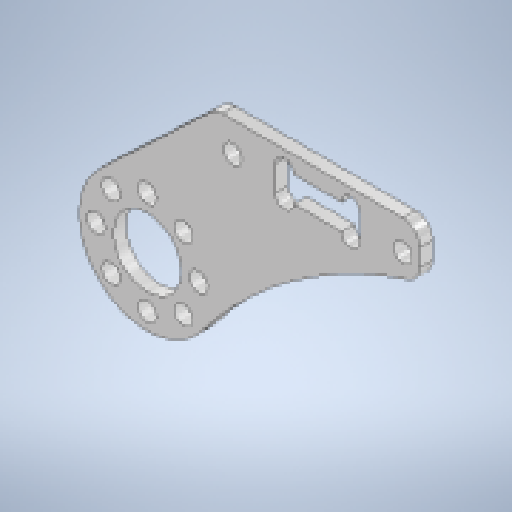
# Autodesk Inventor part: tesaki_new
Saved by Autodesk Inventor 2024 (Build 280153000, 153)
## iProperties
Created: 2023-12-16
Part Number: tesaki_new
Material: アルミニウム 2014-T4
Document SubType Name: Modeling
Designer: right
Density: 2.8 g/cm^3
Appearance: サテン
Mass: 2.30594 g
Surface Area: 15.3884 cm^2
Volume: 0.823551 cm^3
Author: right
Autodesk Inventor part; units mm, degrees
ref_plane "YZ Plane" through (0, 0, 0) normal (1, 0, 0) x (0, 1, 0)
ref_plane "XZ Plane" through (0, 0, 0) normal (0, 1, 0) x (-1, 0, 0)
ref_plane "XY Plane" through (0, 0, 0) normal (0, 0, 1) x (1, 0, 0)
sketch "スケッチ1" plane through (0, 0, 0) normal (0, 0, 1) x (1, 0, 0)
  circle A0 centre (8.8, 8.8) radius 8 projected
  circle A1 centre (2.8, 8.8) radius 0.825 projected
  circle A2 centre (4.5574, 4.5574) radius 0.825 projected
  circle A3 centre (8.8, 2.8) radius 0.825 projected
  circle A4 centre (13.0426, 4.5574) radius 0.825 projected
  circle A5 centre (14.8, 8.8) radius 0.825 projected
  circle A6 centre (13.0426, 13.0426) radius 0.825 projected
  circle A7 centre (8.8, 14.8) radius 0.825 projected
  circle A8 centre (4.5574, 13.0426) radius 0.825 projected
  circle A9 centre (8.8, 8.8) radius 4 projected
  circle A10 centre (8.8, 14.8) radius 1.1
  circle A11 centre (4.5574, 13.0426) radius 1.1
  circle A12 centre (2.8, 8.8) radius 1.1
  circle A13 centre (4.5574, 4.5574) radius 1.1
  circle A14 centre (8.8, 2.8) radius 1.1
  circle A15 centre (13.0426, 4.5574) radius 1.1
  circle A16 centre (14.8, 8.8) radius 1.1
  circle A17 centre (13.0426, 13.0426) radius 1.1
  line L0 (3.3206, 14.6289) -> (16.8, 27.3)
  line L1 (23.8, 25.3) -> (33.8, 25.3)
  line L2 (33.8, 25.3) -> (33.8, 22.3)
  line L3 (33.8, 22.3) -> (23.8, 22.3)
  line L4 (23.8, 22.3) -> (23.8, 25.3)
  circle A18 centre (24.9, 25.3) radius 1.1
  line L5 (28.8, 25.3) -> (28.8, 22.3) construction
  line L6 (28.8, 23.8) -> (23.8, 23.8) construction
  circle A19 centre (24.9, 22.3) radius 1.1
  circle A20 centre (32.7, 25.3) radius 1.1
  circle A21 centre (32.7, 22.3) radius 1.1
  circle A22 centre (38.8, 23.8) radius 1.1
  circle A23 centre (18.8, 23.8) radius 1.1
  line L7 (16.8, 27.3) -> (40.8, 27.3)
  line L8 (40.8, 27.3) -> (40.8, 21.8)
  arc A24 (40.8, 21.8) -> (15.1891, 3.9855) centre (55.1209, -26.1052) ccw
  point P0 (0, 0)
  point P1 (31.6, 22.3)
  point P2 (26, 22.3)
  point P3 (26, 25.3)
  point P4 (31.6, 25.3)
  dimension "d7" = 2.2
  dimension "d0" = 2.2
  dimension "d3" = 360
  dimension "d5" = 10
  dimension "d6" = 3
  dimension "d8" = 2.2
  dimension "d9" = 5
  dimension "d10" = 2
  dimension "d11" = 2
  dimension "d12" = 2
  dimension "d13" = 20
  dimension "d14" = 2
  dimension "d15" = 15
  dimension "d16" = 50
  constraints: 18 end point, 14 centre point, 4 midpoint, 4 point on circle, 4 symmetric about line, 2 horizontal, 2 parallel, 2 tangent, 1 coincident, 1 horizontal alignment, 1 perpendicular, 1 point on line, 1 vertical, 24 other
  measures "d0" diameter of A10
  measures "d5" distance of L2.end L3.end
  measures "d6" distance of L1.end L2.end
  measures "d8" diameter of A22
  measures "d9" distance from line of L4 A23.centre
  measures "d10" distance from line of L7 A20.centre
  measures "d11" distance from line of A22.centre L8
  measures "d12" horizontal distance of L0.end A23.centre
  measures "d13" horizontal distance of A9.centre L6.start
  measures "d14" horizontal distance of L8.end A22.centre
  measures "d15" vertical distance of A9.centre L6.start
  measures "d16" radius of A24
extrude "押し出し1" add sketch "スケッチ1" along normal blind 1.5 contours A0 | A0 L0 L7 L8 A24
fillet "フィレット1" radius 2 3 edges at (40.8, 27.3, 0.75) (40.8, 21.8, 0.75) (16.8, 27.3, 0.75)
sketch "スケッチ4" plane through (0, 0, 0) normal (0, 0, -1) x (-1, 0, 0)
  line L0 (-53.8, 25.3) -> (-43.8, 25.3)
  line L1 (-43.8, 25.3) -> (-43.8, 22.3)
  line L2 (-43.8, 22.3) -> (-53.8, 22.3)
  line L3 (-53.8, 22.3) -> (-53.8, 25.3)
  circle A0 centre (-38.8, 23.8) radius 1.1 projected
  circle A1 centre (-52.7, 25.3) radius 1.1
  line L4 (-48.8, 25.3) -> (-48.8, 23.8) construction
  line L5 (-48.8, 23.8) -> (-53.8, 23.8) construction
  circle A2 centre (-44.9, 25.3) radius 1.1
  circle A3 centre (-52.7, 22.3) radius 1.1
  circle A4 centre (-44.9, 22.3) radius 1.1
  arc A5 (-15.1891, 3.9855) -> (-39.4277, 21.3682) centre (-55.1209, -26.1052) ccw projected
  line L6 (-31.9466, 18.2) -> (-56.8, 18.2)
  line L7 (-56.8, 18.2) -> (-56.8, 27.3)
  line L8 (-38.8, 27.3) -> (-17.5925, 27.3) construction
  line L9 (-56.8, 27.3) -> (-38.8, 27.3)
  arc A6 (-16.2226, 26.7572) -> (-17.5925, 27.3) centre (-17.5925, 25.3) ccw projected
  line L10 (-38.8, 27.3) -> (-17.5925, 27.3) projected
  arc A7 (-38.8, 27.3) -> (-40.8, 25.3) centre (-38.8, 25.3) ccw projected
  line L11 (-40.8, 23.2671) -> (-40.8, 25.3) projected
  arc A8 (-40.8, 23.2671) -> (-39.4277, 21.3682) centre (-38.8, 23.2671) ccw projected
  arc A9 (-15.1891, 3.9855) -> (-39.4277, 21.3682) centre (-55.1209, -26.1052) ccw construction
  arc A10 (-15.1891, 3.9855) -> (-3.3206, 14.6289) centre (-8.8, 8.8) ccw projected
  line L12 (-16.2226, 26.7572) -> (-3.3206, 14.6289) projected
  circle A11 centre (-8.8, 8.8) radius 4 projected
  circle A12 centre (-8.8, 14.8) radius 1.1 projected
  circle A13 centre (-4.5574, 13.0426) radius 1.1 projected
  circle A14 centre (-2.8, 8.8) radius 1.1 projected
  circle A15 centre (-4.5574, 4.5574) radius 1.1 projected
  circle A16 centre (-8.8, 2.8) radius 1.1 projected
  circle A17 centre (-13.0426, 4.5574) radius 1.1 projected
  circle A18 centre (-14.8, 8.8) radius 1.1 projected
  circle A19 centre (-13.0426, 13.0426) radius 1.1 projected
  circle A20 centre (-38.8, 23.8) radius 1.1 projected
  circle A21 centre (-18.8, 23.8) radius 1.1 projected
  line L13 (-33.8, 25.3) -> (-33.8, 22.3) projected
  arc A22 (-31.6, 25.3) -> (-33.8, 25.3) centre (-32.7, 25.3) ccw projected
  line L14 (-26, 25.3) -> (-31.6, 25.3) projected
  arc A23 (-23.8, 25.3) -> (-26, 25.3) centre (-24.9, 25.3) ccw projected
  line L15 (-23.8, 22.3) -> (-23.8, 25.3) projected
  arc A24 (-26, 22.3) -> (-23.8, 22.3) centre (-24.9, 22.3) ccw projected
  line L16 (-31.6, 22.3) -> (-26, 22.3) projected
  arc A25 (-33.8, 22.3) -> (-31.6, 22.3) centre (-32.7, 22.3) ccw projected
  point P0 (0, 0)
  point P1 (-43.8, 23.8)
  point P2 (-39.4277, 21.3682)
  point P3 (-46, 22.3)
  point P4 (-51.6, 22.3)
  point P5 (-51.6, 25.3)
  point P6 (-46, 25.3)
  dimension "d32" = 2.2
  dimension "d30" = 10
  dimension "d31" = 5
  dimension "d33" = 3
  dimension "d34" = 3
  constraints: 18 end point, 3 centre point, 3 horizontal, 3 horizontal alignment, 3 midpoint, 3 symmetric about line, 2 parallel, 2 vertical, 1 perpendicular, 1 point on circle, 1 point on line, 6 other
  measures "d30" distance of L0.start L0.end
  measures "d31" distance of A0.centre point (-43.8, 23.8)
  measures "d33" distance between parallel lines of L7 L3
  measures "d34" distance edge to line of A4 L6
extrude "押し出し4" add sketch "スケッチ4" against normal up to surface (1.5 mm away) contours L6 L7 L9 A7 L11 A8 A5
fillet "フィレット4" radius 4 3 edges at (56.8, 18.2, 0.75) (56.8, 27.3, 0.75) (31.9466, 18.2, 0.75)
